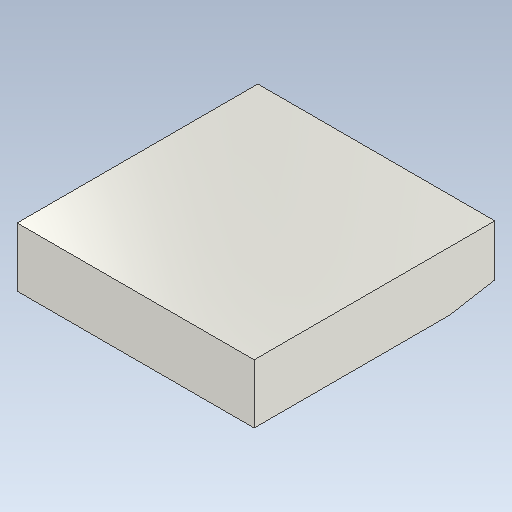
# Autodesk Inventor part: Battery
Saved by Autodesk Inventor 2020 (Build 240168000, 168)
## iProperties
Created: 2021-01-14
Part Number: Battery
Material: Generic
Document SubType Name: Modeling
Designer: Luke
Density: 1 g/cm^3
Appearance: Default
Author: Luke
Autodesk Inventor part; units mm, degrees
ref_plane "Work Plane1" through (43.5156, 8.6766, 49.2201) normal (0, -1, 0) x (-1, 0, 0)
sketch "Sketch1" plane through (43.5156, 8.6766, 49.2201) normal (0, -1, 0) x (-1, 0, 0)
  line L0 (43.0578, -4.3321) -> (72.8078, -4.3321)
  line L1 (72.8078, -4.3321) -> (72.8078, -36.5421)
  line L2 (72.8078, -36.5421) -> (43.0578, -36.5421)
  line L3 (43.0578, -36.5421) -> (43.0578, -4.3321)
  dimension "d0" = 29.75
  dimension "d1" = 32.21
  constraints: 8 end point, 2 parallel, 1 horizontal, 1 perpendicular
  measures "d0" distance of L1.end L2.end
  measures "d1" distance of L0.end L1.end
extrude "Extrusion1" add sketch "Sketch1" along normal blind 7.41
ref_plane "Work Plane2" through (-14.4171, 8.6766, 85.7622) normal (1, 0, 0) x (0, 0, -1)
ref_plane "Work Plane3" through (-29.2921, 1.2666, 53.5522) normal (0, -0.7071, -0.7071) x (1, 0, 0)
sketch "Sketch2" plane through (0.4579, 8.6766, 85.7622) normal (1, 0, 0) x (0, 0, -1)
  line L0 (32.21, 0) -> (30.21, 0)
  line L1 (30.21, 0) -> (30.21, -6.41)
  line L2 (30.21, -7.41) -> (32.21, -7.41)
  line L3 (32.21, -7.41) -> (32.21, 0)
  line L4 (30.21, -6.41) -> (24.5387, -7.41)
  line L5 (24.5387, -7.41) -> (30.21, -7.41)
  constraints: 12 end point, 2 parallel, 1 horizontal, 1 perpendicular
extrude "Extrusion2" cut sketch "Sketch2" against normal through all
body "Solid1"
